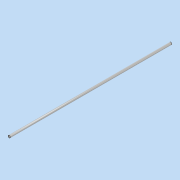
# Autodesk Inventor part: aluminumWiringTubing
Saved by Autodesk Inventor 2017 (Build 210142000, 142)
## iProperties
Created: 2017-04-25
Part Number: aluminumWiringTubing
Material: Aluminum 3003-H14
Document SubType Name: Modeling
Designer: Derek Wider
Mass: 6.66977 g
Surface Area: 88.3322 cm^2
Volume: 2.43592 cm^3
Density: 2.73809 g/cm^3
Appearance: Aluminum - Polished
Author: Derek Wider
Autodesk Inventor part; units mm, degrees
ref_plane "YZ Plane" through (0, 0, 0) normal (1, 0, 0) x (0, 1, 0)
ref_plane "XZ Plane" through (0, 0, 0) normal (0, 1, 0) x (-1, 0, 0)
ref_plane "XY Plane" through (0, 0, 0) normal (0, 0, 1) x (1, 0, 0)
sketch "Sketch1" plane through (0, 0, 0) normal (0, 0, 1) x (1, 0, 0)
  circle A0 centre (0, 0) radius 1.8288
  circle A1 centre (0, 0) radius 2.3813
  dimension "d0" = 3.6576
  dimension "d1" = 4.7625
  constraints: 2 centre point, 2 coincident
  measures "d0" diameter of A0
  measures "d1" diameter of A1
extrude "Extrusion1" add sketch "Sketch1" along normal blind 333.375
body "Solid1"
